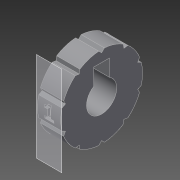
# Autodesk Inventor part: tumbler
Saved by Autodesk Inventor 2017 (Build 210142000, 142)
## iProperties
Created: 2018-04-20
Part Number: tumbler
Material: Generic
Document SubType Name: Modeling
Designer: natha
Density: 1 g/cm^3
Appearance: Default
Author: natha
Autodesk Inventor part; units mm, degrees
ref_plane "YZ Plane" through (0, 0, 0) normal (1, 0, 0) x (0, 1, 0)
ref_plane "XZ Plane" through (0, 0, 0) normal (0, 1, 0) x (-1, 0, 0)
ref_plane "XY Plane" through (0, 0, 0) normal (0, 0, 1) x (1, 0, 0)
sketch "Sketch1" plane through (0, 0, 0) normal (0, 0, 1) x (1, 0, 0)
  line L0 (5.08, -20.2565) -> (0, -20.2565) projected
  line L1 (0, -8.128) -> (33.655, -8.128)
  line L2 (0, -14.478) -> (38.1, -14.478)
  line L3 (0, -8.128) -> (0, -14.478)
  line L4 (0, -11.303) -> (38.1, -11.303)
  line L5 (0, -11.303) -> (5.08, -11.303)
  line L6 (5.08, -11.303) -> (5.08, -20.066)
  line L7 (0, -20.066) -> (0, -11.303)
  circle A0 centre (35.8775, -20.2565) radius 1.27 projected
  circle A1 centre (7.3025, -20.2565) radius 1.27 projected
  line L8 (19.05, -20.2565) -> (19.05, -14.605) projected
  line L9 (19.05, -14.605) -> (14.605, -14.605) projected
  line L10 (14.605, -14.605) -> (14.605, -20.2565) projected
  line L11 (14.605, -20.2565) -> (9.525, -20.2565) projected
  line L12 (9.525, -20.2565) -> (9.525, -14.605) projected
  line L13 (9.525, -14.605) -> (5.08, -14.605) projected
  line L14 (5.08, -14.605) -> (5.08, -20.2565) projected
  line L15 (5.08, -20.2565) -> (0, -20.2565) projected
  line L16 (0, -22.225) -> (0, -20.2565) projected
  line L17 (38.1, -22.225) -> (0, -22.225) projected
  line L18 (38.1, -14.605) -> (38.1, -22.225) projected
  line L19 (38.1, -14.605) -> (33.655, -14.605) projected
  line L20 (33.655, -14.605) -> (33.655, -20.2565) projected
  line L21 (33.655, -20.2565) -> (28.575, -20.2565) projected
  line L22 (28.575, -20.2565) -> (28.575, -14.605) projected
  line L23 (28.575, -14.605) -> (24.13, -14.605) projected
  line L24 (24.13, -14.605) -> (24.13, -20.2565) projected
  line L25 (24.13, -20.2565) -> (19.05, -20.2565) projected
  line L26 (9.525, -11.303) -> (14.605, -11.303)
  line L27 (14.605, -11.303) -> (14.605, -20.2565)
  line L28 (14.605, -20.2565) -> (9.525, -20.2565)
  line L29 (9.525, -20.2565) -> (9.525, -11.303)
  line L30 (19.05, -11.303) -> (24.13, -11.303)
  line L31 (24.13, -11.303) -> (24.13, -20.2565)
  line L32 (24.13, -20.2565) -> (19.05, -20.2565)
  line L33 (19.05, -20.2565) -> (19.05, -11.303)
  line L34 (28.575, -11.303) -> (33.655, -11.303)
  line L35 (33.655, -11.303) -> (33.655, -20.2565)
  line L36 (33.655, -20.2565) -> (28.575, -20.2565)
  line L37 (28.575, -20.2565) -> (28.575, -11.303)
  line L38 (0, -11.303) -> (5.08, -11.303)
  line L39 (5.08, -11.303) -> (5.08, -20.066)
  line L40 (5.08, -20.066) -> (0, -20.066)
  line L41 (0, -20.066) -> (0, -11.303)
  point P0 (0, 0)
  dimension "d14" = 8.763
  constraints: 46 end point, 9 parallel, 8 horizontal, 5 perpendicular, 3 point on line, 2 midpoint, 1 vertical, 4 other
  measures "d14" distance of L6.end L38.end
revolve "Revolution1" add sketch "Sketch1" angle 360 about axis through (0, -11.303, 0) along (1, 0, 0) contours L40 L7 L2 L6 | L2 L3 L4 L6
sketch "Sketch2" plane through (5.08, -11.303, 0) normal (1, 0, 0) x (0, 0, -1)
  arc A0 (-1.5875, 2.7496) -> (1.5875, 2.7496) centre (0, 0) ccw projected
  line L0 (-1.5875, 2.7496) -> (-1.5875, 6.35) projected
  line L1 (1.5875, 6.35) -> (-1.5875, 6.35) projected
  line L2 (1.7145, 2.822) -> (1.7145, 6.477) projected
  arc A1 (0, -3.302) -> (1.7145, 2.822) centre (0, 0) ccw projected
  line L3 (1.7145, 6.477) -> (0, 6.477) projected
  line L4 (0, 3.302) -> (0, 0)
  line L5 (-1.7145, 2.822) -> (-1.7145, 6.477)
  arc A2 (-1.7145, 2.822) -> (0, -3.302) centre (0, 0) ccw
  line L6 (-1.7145, 6.477) -> (0, 6.477)
  line L7 (-1.7145, 6.477) -> (1.7145, 6.477)
  line L8 (1.7145, 6.477) -> (1.7145, 2.822)
  line L9 (-1.7145, 2.822) -> (-1.7145, 6.477)
  arc A3 (-1.7145, 2.822) -> (1.7145, 2.822) centre (0, 0) ccw
  point P0 (0, 11.303)
  constraints: 8 end point, 3 collinear, 2 point on circle, 2 symmetric about line, 1 centre point, 1 coincident, 1 vertical, 1 other
extrude "Extrusion1" cut sketch "Sketch2" against normal through all
sketch "Sketch3" plane through (5.08, -11.303, 0) normal (1, 0, 0) x (0, 0, -1)
  line L0 (-1.7145, 6.477) -> (1.7145, 6.477) projected
  line L1 (1.7145, 6.477) -> (1.7145, 2.822) projected
  arc A0 (-1.7145, 2.822) -> (1.7145, 2.822) centre (0, 0) ccw projected
  line L2 (-1.7145, 2.822) -> (-1.7145, 6.477) projected
  line L3 (0, 8.6897) -> (0, 7.6061)
  circle A1 centre (0, 0) radius 8.763 projected
  line L4 (0, 8.128) -> (0.6135, 8.7415)
  line L5 (0, 8.128) -> (0.8676, 8.128) construction
  line L6 (0, 8.128) -> (-0.6009, 8.7424)
  arc A2 (0.6135, 8.7415) -> (-0.6009, 8.7424) centre (0, 0) ccw
  arc A3 (-4.6418, 7.4326) -> (-5.6247, 6.7196) centre (0, 0) ccw
  line L7 (-4.7775, 6.5757) -> (-5.6247, 6.7196)
  line L8 (-4.7775, 6.5757) -> (-4.6418, 7.4326)
  arc A4 (-8.1241, 3.2847) -> (-8.5002, 2.1301) centre (0, 0) ccw
  line L9 (-7.7302, 2.5117) -> (-8.5002, 2.1301)
  line L10 (-7.7302, 2.5117) -> (-8.1241, 3.2847)
  arc A5 (-8.5032, -2.1178) -> (-8.1288, -3.273) centre (0, 0) ccw
  line L11 (-7.7302, -2.5117) -> (-8.1288, -3.273)
  line L12 (-7.7302, -2.5117) -> (-8.5032, -2.1178)
  arc A6 (-5.6345, -6.7114) -> (-4.6525, -7.4259) centre (0, 0) ccw
  line L13 (-4.7775, -6.5757) -> (-4.6525, -7.4259)
  line L14 (-4.7775, -6.5757) -> (-5.6345, -6.7114)
  arc A7 (-0.6135, -8.7415) -> (0.6009, -8.7424) centre (0, 0) ccw
  line L15 (0, -8.128) -> (0.6009, -8.7424)
  line L16 (0, -8.128) -> (-0.6135, -8.7415)
  arc A8 (4.6418, -7.4326) -> (5.6247, -6.7196) centre (0, 0) ccw
  line L17 (4.7775, -6.5757) -> (5.6247, -6.7196)
  line L18 (4.7775, -6.5757) -> (4.6418, -7.4326)
  arc A9 (8.1241, -3.2847) -> (8.5002, -2.1301) centre (0, 0) ccw
  line L19 (7.7302, -2.5117) -> (8.5002, -2.1301)
  line L20 (7.7302, -2.5117) -> (8.1241, -3.2847)
  arc A10 (8.5032, 2.1178) -> (8.1288, 3.273) centre (0, 0) ccw
  line L21 (7.7302, 2.5117) -> (8.1288, 3.273)
  line L22 (7.7302, 2.5117) -> (8.5032, 2.1178)
  arc A11 (5.6345, 6.7114) -> (4.6525, 7.4259) centre (0, 0) ccw
  line L23 (4.7775, 6.5757) -> (4.6525, 7.4259)
  line L24 (4.7775, 6.5757) -> (5.6345, 6.7114)
  point P0 (0, 11.303)
  point P1 (0, 8.763)
  dimension "d3" = 0.635
  dimension "d4" = 45
  dimension "d7" = 360
  constraints: 44 end point, 23 point on circle, 10 centre point, 2 point on line, 1 coincident, 1 equal length, 1 horizontal, 1 vertical, 71 other
  measures "d3" distance of L4.start A1.start
  measures "d4" angle of L5 L4
extrude "Extrusion2" cut sketch "Sketch3" against normal through all contours L22 L21 A1 | A1 L20 L19 | L24 L23 A1 | A1 L18 L17 | L4 L6 A1 | A1 L16 L15 | L8 L7 A1 | A1 L14 L13 | L10 L9 A1 | A1 L12 L11
ref_plane "Work Plane2" through (2.54, -11.303, 8.763) normal (0, 0, 1) x (1, 0, 0)
sketch "Sketch5" plane through (2.54, -11.303, 8.763) normal (0, 0, 1) x (1, 0, 0)
  line L0 (-1.4457, 1.5835) -> (1.4569, 1.5835) construction
  line L1 (1.4569, 1.5835) -> (1.4569, -1.4719) construction
  line L2 (1.4569, -1.4719) -> (-1.4457, -1.4719) construction
  line L3 (-1.4457, -1.4719) -> (-1.4457, 1.5835) construction
  line L4 (0.9675, -1.4719) -> (-1.0456, -1.4719)
  line L5 (-1.0456, -1.4719) -> (-1.0456, -0.9408)
  line L6 (-1.0456, -0.9408) -> (-0.4034, -0.9408)
  line L7 (-0.4034, -0.9408) -> (-0.4034, 0.6721)
  line L8 (-0.4034, 0.6721) -> (-1.0456, 0.6721)
  line L9 (-1.0456, 0.6721) -> (-1.0456, 1.1686)
  spline S0 degree 2 poles (-1.0456, 1.1686) (-0.9048, 1.1686) (-0.6257, 1.2056) (-0.5417, 1.2451) knots 0 0 0 1 2 2 2
  spline S1 degree 2 poles (-0.5417, 1.2451) (-0.4454, 1.2945) (-0.3367, 1.46) (-0.3268, 1.5835) knots 0 0 0 1 2 2 2
  line L10 (-0.3268, 1.5835) -> (0.3401, 1.5835)
  line L11 (0.3401, 1.5835) -> (0.3401, -0.9408)
  line L12 (0.3401, -0.9408) -> (0.9675, -0.9408)
  line L13 (0.9675, -0.9408) -> (0.9675, -1.4719)
  point P0 (-2.54, 11.303)
  constraints: 2 other
emboss "Emboss2" sketch "Sketch5" operation cut depth 0.635 direction (0, 0, -1) wrap yes faces at (1.6933, -12.9553, 8.6058)
body "Solid1"
